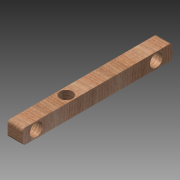
# Autodesk Inventor part: legrod
Saved by Autodesk Inventor 2015 (Build 190159000, 159)
## iProperties
Created: 2020-01-20
Part Number: legrod
Material: Wood (Birch)
Document SubType Name: Modeling
Designer: hp
Density: 0.55 g/cm^3
Appearance: Birch - Natural Polished
Author: hp
Autodesk Inventor part; units mm, degrees
ref_plane "YZ Plane" through (0, 0, 0) normal (1, 0, 0) x (0, 1, 0)
ref_plane "XZ Plane" through (0, 0, 0) normal (0, 1, 0) x (-1, 0, 0)
ref_plane "XY Plane" through (0, 0, 0) normal (0, 0, 1) x (1, 0, 0)
sketch "Sketch1" plane through (0, 0, 0) normal (1, 0, 0) x (0, 1, 0)
  line L0 (0.9972, 8.0994) -> (0.9972, -18.9664)
  line L1 (0.9972, -18.9664) -> (0.9972, 581.0324)
  line L2 (0.9972, 581.0324) -> (60.997, 581.0324)
  line L3 (60.997, 581.0324) -> (60.997, -18.9664)
  line L4 (60.997, -18.9664) -> (0.9972, -18.9664)
  point P0 (0, 0)
  dimension "d0" = 599.9988
  dimension "d1" = 59.9999
  constraints: 10 end point, 3 perpendicular, 1 point on line, 1 vertical
  measures "d0" distance of L0.end L1.end
  measures "d1" distance of L1.end L2.end
extrude "Extrusion1" add sketch "Sketch1" along normal blind 59.9948
sketch "Sketch2" plane through (59.9948, 0, 0) normal (1, 0, 0) x (0, 0, -1)
  circle A0 centre (-525.9231, 30.9971) radius 25.4
  circle A1 centre (-45.3472, 30.9971) radius 25.4
  point P0 (0, 0)
  dimension "d4" = 50.8
  dimension "d5" = 50.8
  constraints: 2 centre point
  measures "d4" diameter of A0
  measures "d5" diameter of A1
extrude "Extrusion2" cut sketch "Sketch2" against normal blind 59.9948
fillet "Fillet1" radius 12.7 4 edges at (29.9974, 60.997, 581.0324) (29.9974, 0.9972, 581.0324) (29.9974, 60.997, -18.9664) (29.9974, 0.9972, -18.9664)
sketch "Sketch3" plane through (0, 60.997, 568.3324) normal (0, 1, 0) x (1, 0, 0)
  circle A0 centre (29.9562, 192.5093) radius 25.4
  point P0 (0, 568.3324)
  dimension "d9" = 50.8
  constraints: 1 centre point
  measures "d9" diameter of A0
extrude "Extrusion3" cut sketch "Sketch3" against normal blind 50.8
body "Solid1"
